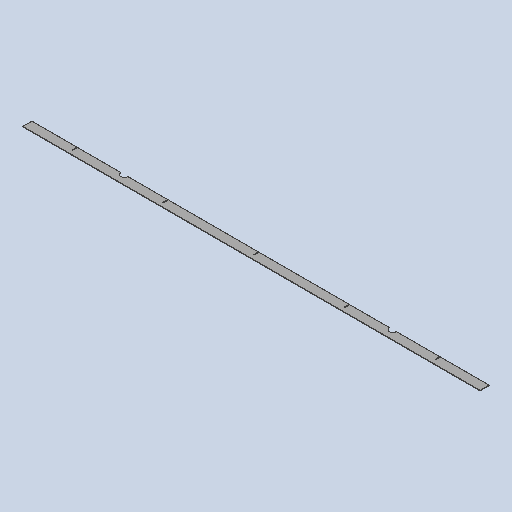
# Autodesk Inventor part: BSH 024 stringer floor
Saved by Autodesk Inventor 2025 (Build 290162010, 162A)
## iProperties
Created: 2024-07-23
Part Number: BSH 024 stringer floor
Material: 09g2s
Document SubType Name: Sheet Metal
Designer: pokla
Mass: 5330.4 g
Surface Area: 4696.25 cm^2
Volume: 679.031 cm^3
Density: 7.85 g/cm^3
Flat Pattern Width: 5 cm
Flat Pattern Length: 252 cm
Flat Pattern Area: 1260 cm^2
Sheet Metal Rule: AISI304 3mm Die 32
Sheet Metal Width: 50,000 mm
Sheet Metal Length: 2520,000 mm
Sheet Metal Area: 126000,000 mm^2
Appearance: Default
Author: admin
Autodesk Inventor part; units mm, degrees
ref_plane "YZ Plane" through (0, 0, 0) normal (1, 0, 0) x (0, 1, 0)
ref_plane "XZ Plane" through (0, 0, 0) normal (0, 1, 0) x (-1, 0, 0)
ref_plane "XY Plane" through (0, 0, 0) normal (0, 0, 1) x (1, 0, 0)
sketch "Sketch8" plane through (0, 0, 0) normal (0, 0, 1) x (1, 0, 0)
  line L0 (-1260, 50) -> (1260, 50)
  line L1 (1260, 50) -> (1260, 0)
  line L2 (1260, 0) -> (-1260, 0)
  line L3 (-1260, 0) -> (-1260, 50)
  point P0 (0, 0)
  point P1 (0, 0)
  dimension "d37" = 50
  dimension "d38" = 2520
  measures "d37" distance of L2.end L0.start
  measures "d38" distance of L0.start L0.end
extrude "Plate5" add sketch "Sketch8" against normal blind 3
sketch "Sketch9" plane through (0, 0, 0) normal (0, 0, 1) x (1, 0, 0)
  line L0 (1260, 50) -> (-1260, 50) projected
  line L1 (-1011.6, 50) -> (-1008.4, 50)
  line L2 (-1008.4, 50) -> (-1008.4, 24)
  line L3 (-1008.4, 24) -> (-1011.6, 24)
  line L4 (-1011.6, 24) -> (-1011.6, 50)
  point P0 (0, 0)
  point P1 (-1008.4, 50)
  dimension "d40" = 248.4
  dimension "d41" = 3.2
  dimension "d42" = 26
  constraints: 8 end point, 2 parallel, 1 horizontal, 1 perpendicular, 1 point on line
  measures "d40" distance of L1.start L0.end
  measures "d41" distance between parallel lines of L4 L2
  measures "d42" distance of L1.end L2.end
extrude "Extrusion3" cut sketch "Sketch9" against normal through all
pattern_linear "Rectangular Pattern2" count 5 spacing 500 along (1, 0, 0) of "Extrusion3"
sketch "Sketch10" plane through (0, 0, -3) normal (0, 0, -1) x (-1, 0, 0)
  line L0 (-988.4, 50) -> (-988.4, 24) projected
  line L1 (-988.4, 24) -> (-991.6, 24) projected
  line L2 (-991.6, 24) -> (-991.6, 50) projected
  line L3 (-1260, 50) -> (-991.6, 50) projected
  line L4 (-1260, 0) -> (-1260, 50) projected
  line L5 (1260, 0) -> (-1260, 0) projected
  line L6 (1260, 50) -> (1260, 0) projected
  line L7 (1011.6, 50) -> (1260, 50) projected
  line L8 (1011.6, 50) -> (1011.6, 24) projected
  line L9 (1011.6, 24) -> (1008.4, 24) projected
  line L10 (1008.4, 24) -> (1008.4, 50) projected
  line L11 (511.6, 50) -> (1008.4, 50) projected
  line L12 (511.6, 50) -> (511.6, 24) projected
  line L13 (511.6, 24) -> (508.4, 24) projected
  line L14 (508.4, 24) -> (508.4, 50) projected
  line L15 (11.6, 50) -> (508.4, 50) projected
  line L16 (11.6, 50) -> (11.6, 24) projected
  line L17 (11.6, 24) -> (8.4, 24) projected
  line L18 (8.4, 24) -> (8.4, 50) projected
  line L19 (-488.4, 50) -> (8.4, 50) projected
  line L20 (-488.4, 50) -> (-488.4, 24) projected
  line L21 (-488.4, 24) -> (-491.6, 24) projected
  line L22 (-491.6, 24) -> (-491.6, 50) projected
  line L23 (-988.4, 50) -> (-491.6, 50) projected
  circle A0 centre (750, 50) radius 20
  line L24 (11.6, 50) -> (508.4, 50) projected
  circle A1 centre (-730, 50) radius 20
  point P0 (0, 0)
  point P1 (770, 50)
  point P2 (730, 50)
  point P3 (-710, 50)
  point P4 (-750, 50)
  dimension "d48" = 40
  dimension "d49" = 40
  dimension "d50" = 1480
  dimension "d51" = 530
  constraints: 3 point on line, 2 centre point
  measures "d48" diameter of A0
  measures "d49" diameter of A1
  measures "d50" distance of A0.centre A1.centre
  measures "d51" distance from line of L4 A1.centre
extrude "Extrusion4" cut sketch "Sketch10" against normal through all contours L23 A1 | A0 L11 picked at (-735.7537, 42.481) picked at (744.2463, 42.481)
equation "\"d39\" = Thickness"
equation "\"BendReliefWidth\" = Thickness"
equation "\"BendReliefDepth\" = 0.5 * Thickness"
equation "\"CornerReliefSize\" = 4 * Thickness"
equation "\"MinimumRemnant\" = 2 * Thickness"
equation "\"TransitionRadius\" = BendRadius"
equation "\"JacobiRadiusSize\" = BendRadius"
equation "\"GapSize\" = Thickness"
equation "\"Thickness\" = 3"
equation "\"BendRadius\" = 5"
body "Solid3"
